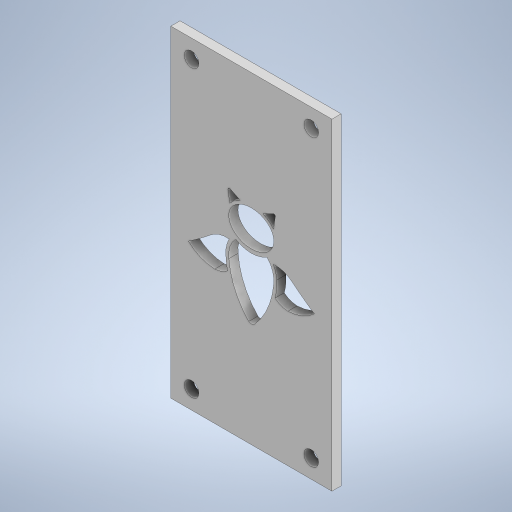
# Autodesk Inventor part: lid
Saved by Autodesk Inventor 2024 (Build 280153000, 153)
## iProperties
Created: 2023-11-10
Part Number: lid
Material: 一般
Document SubType Name: Modeling
Designer: Kota Taga
Density: 1 g/cm^3
Appearance: 既定
Author: Kota Taga
## iProperties of the stored document lid_3D プリント.ipt
Created: 2023-11-10
Part Number: lid_3D プリント
Material: 一般
Document SubType Name: Modeling
Designer: Kota Taga
Density: 1 g/cm^3
Appearance: 既定
Author: Kota Taga
Autodesk Inventor part; units mm, degrees
ref_plane "YZ Plane" through (0, 0, 0) normal (1, 0, 0) x (0, 1, 0)
ref_plane "XZ Plane" through (0, 0, 0) normal (0, 1, 0) x (-1, 0, 0)
ref_plane "XY Plane" through (0, 0, 0) normal (0, 0, 1) x (1, 0, 0)
sketch "スケッチ1" plane through (0, 0, 0) normal (0, 0, 1) x (1, 0, 0)
  line L0 (-19.75, 35) -> (19.75, 35)
  line L1 (19.75, 35) -> (19.75, -35)
  line L2 (19.75, -35) -> (-19.75, -35)
  line L3 (-19.75, -35) -> (-19.75, 35)
  line L4 (-27.65, 0) -> (27.65, 0) projected
  line L5 (0, -49) -> (0, 49) projected
  point P0 (0, 0)
  dimension "d0" = 39.5
  dimension "d1" = 70
  constraints: 8 end point, 2 parallel, 1 horizontal, 1 perpendicular, 2 other
  measures "d0" distance of L0.start L0.end
  measures "d1" distance of L0.end L1.end
extrude "押し出し1" add sketch "スケッチ1" along normal blind 2
sketch "スケッチ2" plane through (0, 0, 2) normal (0, 0, 1) x (1, 0, 0)
  line L0 (19.75, 35) -> (-19.75, 35) projected
  line L1 (-19.75, 35) -> (70.2885, 35) construction
  line L2 (70.2885, 35) -> (70.2885, -4.6911) construction
  line L3 (70.2885, -4.6911) -> (-19.75, -4.6911) construction
  line L4 (-19.75, -4.6911) -> (-19.75, 35) construction
  line L5 (-19.75, -35) -> (19.75, -35) projected
  point P0 (0, 0)
  dimension "d24" = 30.3089
  constraints: 2 other
  measures "d24" distance between parallel lines of L5 L3
sketch "スケッチ3" plane through (0, 0, 2) normal (0, 0, 1) x (1, 0, 0)
  arc A0 (-3.4095, 1.9716) -> (3.3759, 1.9716) centre (-0.0168, 7.4667) ccw
  arc A1 (-2.4389, 9.7787) -> (-4.7032, 8.0756) centre (-0.3535, 4.6495) ccw
  arc A2 (4.7988, 7.9483) -> (2.4955, 9.7159) centre (0.732, 5.0335) ccw
  arc A3 (-4.6829, 10.8815) -> (-5.087, 10.5506) centre (-4.7267, 10.5227) ccw
  line L0 (-5.087, 10.5506) -> (-4.7032, 8.0756)
  line L1 (-4.6829, 10.8815) -> (-2.4389, 9.7787)
  arc A4 (5.2, 10.5955) -> (4.8431, 10.8815) centre (4.8669, 10.5454) ccw
  line L2 (5.2, 10.5955) -> (4.7988, 7.9483)
  line L3 (2.4955, 9.7159) -> (4.8431, 10.8815)
  ellipse E0 centre (-0.0168, 5.6987) end of major axis (-0.0168, 9.5622) minor radius 4.9125
  arc A5 (-3.4095, 1.9716) -> (-4.8951, -2.438) centre (0.3318, -1.7439) ccw
  arc A6 (-4.8951, -2.438) -> (-0.5921, -12.1143) centre (10.9649, -1.1801) ccw
  arc A7 (-0.5921, -12.1143) -> (0.5903, -12.1143) centre (-0.0009, -11.1325) ccw
  arc A8 (0.5903, -12.1143) -> (4.8431, -2.438) centre (-11.633, -0.9693) ccw
  arc A9 (4.8431, -2.438) -> (3.3759, 1.9716) centre (-0.3664, -1.7225) ccw
  arc A10 (-13.6829, -3.5408) -> (-8.9969, -0.0623) centre (-49.5985, 49.739) ccw
  arc A11 (-4.8311, 1.2871) -> (-8.9969, -0.0623) centre (-5.3873, -4.1006) ccw
  arc A12 (-4.8311, 1.2871) -> (-5.5346, -2.0499) centre (0.4254, -1.5637) ccw
  arc A13 (-5.5346, -2.0499) -> (-5.1537, -4.8603) centre (5.3624, -2.004) ccw
  arc A14 (-13.6829, -3.5408) -> (-7.9463, -5.9228) centre (-7.6688, 2.8445) ccw
  arc A15 (-7.9463, -5.9228) -> (-5.1537, -4.8603) centre (-8.0736, -1.3869) ccw
  line L4 (-0.3527, 5.2511) -> (-0.3527, -27.0056)
  arc A16 (8.9799, -0.0623) -> (13.666, -3.5408) centre (49.5815, 49.739) ccw
  arc A17 (8.9799, -0.0623) -> (4.7845, 1.3168) centre (5.3378, -4.0712) ccw
  arc A18 (5.5023, -1.2772) -> (4.7845, 1.3168) centre (-0.472, -1.534) ccw
  arc A19 (5.1368, -4.8603) -> (5.5023, -1.2772) centre (-5.409, -1.9744) ccw
  arc A20 (7.9294, -5.9228) -> (13.666, -3.5408) centre (7.6518, 2.8445) ccw
  arc A21 (5.1368, -4.8603) -> (7.9294, -5.9228) centre (8.0567, -1.3869) ccw
  line L5 (-19.75, -35) -> (19.75, -35) projected
  line L6 (19.75, 35) -> (-19.75, 35) projected
  line L7 (19.75, -35) -> (19.75, 35) projected
  line L8 (-19.75, 35) -> (-19.75, -35) projected
  point P0 (0, 0)
  point P1 (3.7782, 9.0029)
  point P2 (5.2, 10.5955)
  dimension "d27" = 1.768
  dimension "d28" = 1.0492
  dimension "d29" = 3.3042
  dimension "d30" = 29.3013
  dimension "d31" = 9.7993
  dimension "d46" = 6.084
  constraints: 46 point on circle, 22 centre point, 10 end point, 1 vertical, 2 other
  measures "d27" distance of A0.centre point (-0.017, 5.699)
  measures "d28" vertical distance of point (-0.017, 5.699) A1.centre
  measures "d29" vertical distance of point (-0.017, 5.699) point (3.778, 9.003)
  measures "d30" distance from line of L6 point (-0.017, 5.699)
  measures "d31" vertical distance of A11.centre point (-0.017, 5.699)
  measures "d46" distance from line of L7 A16.end
extrude "押し出し2" cut sketch "スケッチ3" against normal up to surface (2 mm away) contours E0 | A0 L4 A7 A6 A5 | A0 A9 A8 A7 L4 | A1 L0 A3 L1 | A2 L3 A4 L2 | A10 A11 A12 A13 A15 A14 | A16 A20 A21 A19 A18 A17
sketch "スケッチ4" plane through (0, 0, 2) normal (0, 0, 1) x (1, 0, 0)
  circle A0 centre (-13, 31) radius 1.6
  line L0 (19.75, 35) -> (-19.75, 35) projected
  line L1 (-19.75, 35) -> (-19.75, -35) projected
  line L2 (-37.7577, 0) -> (88.2962, 0) projected
  line L3 (0, -49) -> (0, 49) projected
  circle A1 centre (13, 31) radius 1.6
  circle A2 centre (-13, -31) radius 1.6
  circle A3 centre (13, -31) radius 1.6
  point P0 (0, 0)
  dimension "d35" = 4
  dimension "d37" = 3.2
  dimension "d49" = 26
  constraints: 4 centre point, 3 symmetric about line, 3 other
  measures "d35" distance from line of L0 A0.centre
  measures "d37" diameter of A0
  measures "d49" distance of A1.centre A0.centre
extrude "押し出し3" cut sketch "スケッチ4" against normal up to surface (2 mm away) contours A0 | A1 | A2 | A3
sketch "スケッチ5" plane through (0, 0, 2) normal (0, 0, 1) x (1, 0, 0)
  line L0 (-19.75, 35) -> (-19.75, -35) projected
  line L1 (-19.75, 35) -> (-20.75, 35)
  line L2 (-20.75, 35) -> (-20.75, -35)
  line L3 (-20.75, -35) -> (-19.75, -35)
  line L4 (-19.75, -35) -> (-19.75, 35)
  line L5 (19.75, -35) -> (19.75, 35) projected
  line L6 (19.75, 35) -> (20.75, 35)
  line L7 (20.75, 35) -> (20.75, -35)
  line L8 (20.75, -35) -> (19.75, -35)
  line L9 (19.75, -35) -> (19.75, 35)
  point P0 (0, 0)
  dimension "d40" = 1
  dimension "d41" = 1
  constraints: 16 end point, 4 parallel, 2 horizontal, 2 perpendicular, 1 point on line
  measures "d40" distance of L3.end L2.end
  measures "d41" distance of L7.end L8.end
extrude "押し出し4" add sketch "スケッチ5" against normal up to surface (2 mm away)
sketch "スケッチ6" plane through (0, 0, 2) normal (0, 0, 1) x (1, 0, 0)
  line L0 (-12, 12) -> (12, 12)
  line L1 (12, 12) -> (12, -12)
  line L2 (12, -12) -> (-12, -12)
  line L3 (-12, -12) -> (-12, 12)
  line L4 (-38.9577, 0) -> (88.4962, 0) projected
  line L5 (0, -49) -> (0, 49) projected
  point P0 (0, 0)
  dimension "d44" = 24
  dimension "d45" = 24
  constraints: 8 end point, 2 parallel, 1 horizontal, 1 perpendicular, 2 other
  measures "d44" distance of L1.end L2.end
  measures "d45" distance of L0.end L1.end
sketch "スケッチ7" plane through (0, 0, 2) normal (0, 0, 1) x (1, 0, 0)
  line L0 (20.75, 35) -> (-20.75, 35) projected
  line L1 (-20.75, -35) -> (20.75, -35) projected
  line L2 (-17.5, 35) -> (17.5, 35)
  line L3 (17.5, 35) -> (17.5, -35)
  line L4 (17.5, -35) -> (-17.5, -35)
  line L5 (-17.5, -35) -> (-17.5, 35)
  line L6 (-38.9577, 0) -> (88.4962, 0) projected
  line L7 (0, -49) -> (0, 49) projected
  line L8 (-20.75, 35) -> (-20.75, -35) projected
  line L9 (-17.5, 35) -> (-20.75, 35)
  line L10 (-20.75, 35) -> (-20.75, -35)
  line L11 (-20.75, -35) -> (-17.5, -35)
  line L12 (-17.5, -35) -> (-17.5, 35)
  line L13 (17.5, -35) -> (20.75, -35)
  line L14 (20.75, -35) -> (20.75, 35)
  line L15 (20.75, 35) -> (17.5, 35)
  line L16 (17.5, 35) -> (17.5, -35)
  point P0 (0, 0)
  point P1 (20.75, -35)
  dimension "d50" = 35
  constraints: 24 end point, 6 parallel, 3 horizontal, 3 perpendicular, 2 point on line, 1 other
  measures "d50" distance between parallel lines of L3 L5
extrude "押し出し5" cut sketch "スケッチ7" against normal up to surface (2 mm away) contours L14 L6 L3 L0 | L14 L1 L3 L6 | L5 L6 L8 L0 | L5 L1 L8 L6
